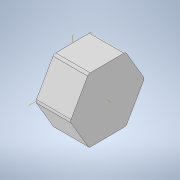
# Autodesk Inventor part: crank case
Saved by Autodesk Inventor 2021.1 (Build 251245000, 245)
## iProperties
Created: 2020-08-29
Part Number: crank case
Material: Generic
Document SubType Name: Sheet Metal
Designer: Vamshi
Density: 1 g/cm^3
Sheet Metal Rule: Default
Appearance: Default
Author: Vamshi
Autodesk Inventor part; units mm, degrees
ref_plane "YZ Plane" through (0, 0, 0) normal (1, 0, 0) x (0, 1, 0)
ref_plane "XZ Plane" through (0, 0, 0) normal (0, 1, 0) x (-1, 0, 0)
ref_plane "XY Plane" through (0, 0, 0) normal (0, 0, 1) x (1, 0, 0)
sketch "Sketch1" plane through (0, 0, 0) normal (0, 0, 1) x (1, 0, 0)
  line L0 (71.3654, -134.1058) -> (-69.412, -135.1271)
  line L1 (-80.4563, -128.8571) -> (-151.7295, -7.451)
  line L2 (-151.8217, 5.2487) -> (-82.3175, 127.6761)
  line L3 (-71.3654, 134.1058) -> (69.412, 135.1271)
  line L4 (80.4563, 128.8571) -> (151.7295, 7.451)
  line L5 (151.8217, -5.2487) -> (82.3175, -127.6761)
  arc A0 (-71.3654, 134.1058) -> (-82.3175, 127.6761) centre (-71.2732, 121.4061) ccw
  arc A1 (80.4563, 128.8571) -> (69.412, 135.1271) centre (69.5041, 122.4275) ccw
  arc A2 (151.8217, -5.2487) -> (151.7295, 7.451) centre (140.7774, 1.0214) ccw
  arc A3 (71.3654, -134.1058) -> (82.3175, -127.6761) centre (71.2732, -121.4061) ccw
  arc A4 (-80.4563, -128.8571) -> (-69.412, -135.1271) centre (-69.5041, -122.4275) ccw
  arc A5 (-151.8217, 5.2487) -> (-151.7295, -7.451) centre (-140.7774, -1.0214) ccw
  point P0 (0, 0)
  point P1 (0, 0)
  point P2 (78.6975, -134.0526)
  point P3 (-76.7442, -135.1803)
  point P4 (-155.4417, -1.1278)
  point P5 (-78.6975, 134.0526)
  point P6 (76.7442, 135.1803)
  point P7 (155.4417, 1.1278)
  dimension "d0" = 269.24
  dimension "d1" = 12.7
  constraints: 12 end point, 12 point on circle, 12 point on line, 12 tangent, 6 centre point, 5 equal radius, 1 coincident, 13 other
  measures "d0" distance between parallel lines of L0 L3
  measures "d1" radius of A0
extrude "Extrusion1" add sketch "Sketch1" along normal blind 144.78
equation "\"BendRadius\" = Thickness"
equation "\"BendReliefWidth\" = Thickness"
equation "\"BendReliefDepth\" = 0.5 * Thickness"
equation "\"CornerReliefSize\" = 4 * Thickness"
equation "\"MinimumRemnant\" = 2 * Thickness"
equation "\"TransitionRadius\" = BendRadius"
equation "\"JacobiRadiusSize\" = BendRadius"
equation "\"GapSize\" = Thickness"
equation "\"Thickness\" = 3.048"
body "Solid1"
